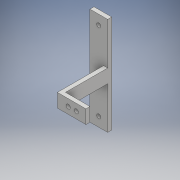
# Autodesk Inventor part: soporteOdroid
Saved by Autodesk Inventor 2017 (Build 210142000, 142)
## iProperties
Part Number: soporteOdroid
Material: Genérico
Document SubType Name: Modeling
Designer: Roberto
Density: 1 g/cm^3
Appearance: Valor por defecto
Author: Roberto
Autodesk Inventor part; units mm, degrees
ref_plane "YZ Plane" through (0, 0, 0) normal (1, 0, 0) x (0, 1, 0)
ref_plane "XZ Plane" through (0, 0, 0) normal (0, 1, 0) x (-1, 0, 0)
ref_plane "XY Plane" through (0, 0, 0) normal (0, 0, 1) x (1, 0, 0)
sketch "Boceto1" plane through (0, 0, 0) normal (0, 1, 0) x (-1, 0, 0)
  circle A0 centre (0.65, -0.45) radius 0.15
  line L0 (0.3, 0) -> (1.3, 0)
  line L1 (1.3, 0) -> (1.3, -1)
  line L2 (1.3, -1) -> (0.3, -1)
  line L3 (0.3, -1) -> (0, -1)
  line L4 (0, -1) -> (0, 0)
  line L5 (0, 0) -> (0.3, 0)
  constraints: 12 end point, 1 centre point
extrude "Extrusión1" add sketch "Boceto1" along normal blind 0.3
sketch "Boceto2" plane through (0, 0, 0) normal (0, -1, 0) x (1, 0, 0)
  line L0 (0, -1) -> (0, 0)
  line L1 (-0.3, -1) -> (0, -1)
  line L2 (0, 0) -> (-0.3, 0)
  line L3 (-0.3, 0) -> (-0.3, -1)
  line L4 (0, 0) -> (0, -1) projected
  line L5 (-0.3, -1) -> (0, -1)
  line L6 (0, -1) -> (0, 0)
  line L7 (0, 0) -> (-0.3, 0)
  line L8 (-0.3, 0) -> (-0.3, -1)
  constraints: 16 end point, 2 parallel, 1 horizontal, 1 perpendicular
extrude "Extrusión2" add sketch "Boceto2" along normal blind 3.4
sketch "Boceto3" plane through (0, 0.3, 0) normal (1, 0, 0) x (0, 0, -1)
  line L0 (1, 0) -> (1, -3.7) projected
  line L1 (0, 0) -> (1, 0) projected
  line L2 (0, 0) -> (0, -3.7) projected
  line L3 (1, -3.7) -> (0, -3.7) projected
  line L4 (0, 0) -> (0, -3.7) projected
  line L5 (0, -3.7) -> (0, -3.4)
  line L6 (0, -3.4) -> (1, -3.4)
  line L7 (1, -3.4) -> (1, -3.7)
  line L8 (1, -3.7) -> (0, -3.7)
  line L9 (0, -3.7) -> (0, -3.4)
  point P0 (0, -0.3)
  dimension "d4" = 0.3
  constraints: 10 end point, 2 parallel, 1 horizontal, 1 perpendicular, 1 point on line
  measures "d4" distance of L2.end L5.end
extrude "Extrusión3" add sketch "Boceto3" along normal blind 1.8 contours L0 L3 L2 L6
sketch "Boceto4" plane through (0, -3.4, 0) normal (0, -1, 0) x (1, 0, 0)
  line L0 (-0.3, 0) -> (1.8, 0) projected
  line L1 (-0.3, 0) -> (-0.3, -1) projected
  line L2 (-0.3, -1) -> (1.8, -1) projected
  line L3 (1.8, 0) -> (1.8, -1) projected
  circle A0 centre (0.5, -0.5) radius 0.15
  circle A1 centre (-6.552, -4.409) radius 0.15
  circle A2 centre (-5.952, -4.409) radius 0.15
  line L4 (0.5, -0.5) -> (1.1, -0.5)
  circle A3 centre (1.1, -0.5) radius 0.15
  point P0 (0, 0)
  dimension "d7" = 0.3
  dimension "d18" = 0.3
  dimension "d19" = 0.3
  dimension "d21" = 0.3
  constraints: 4 centre point, 2 end point, 1 coincident, 1 horizontal
  measures "d7" diameter of A0
  measures "d18" diameter of A1
  measures "d19" diameter of A2
  measures "d21" diameter of A3
extrude "Extrusión4" cut sketch "Boceto4" against normal blind 1 contours A0 | A3
sketch "Boceto6" plane through (0, 0.3, 0) normal (0, 1, 0) x (1, 0, 0)
  line L0 (-1.3, 1) -> (-1.3, 0) projected
  line L1 (-1.3, 0.5) -> (-1.3, 3.4)
  line L2 (0, 3.4) -> (0, -2.4)
  line L3 (-1.3, -2.4) -> (-1.3, 0.5)
  circle A0 centre (-0.65, -2.4) radius 0.15
  circle A1 centre (-0.65, 3.4) radius 0.15
  line L4 (0, 3.4) -> (0, 4.1)
  line L5 (0, 4.1) -> (-1.3, 4.1)
  line L6 (-1.3, 4.1) -> (-1.3, 3.4)
  line L7 (-1.3, -2.4) -> (-1.3, -3.1)
  line L8 (-1.3, -3.1) -> (0, -3.1)
  line L9 (0, -3.1) -> (0, -2.4)
  point P0 (0, 0)
  dimension "d22" = 2.9
  dimension "d23" = 5.8
  dimension "d24" = 1.3
  dimension "d25" = 0.3
  dimension "d26" = 0.3
  dimension "d28" = 0.7
  constraints: 18 end point, 3 perpendicular, 3 point on line, 2 centre point, 2 vertical, 1 collinear, 1 midpoint
  measures "d22" distance of L1.start L1.end
  measures "d23" distance of L2.start L2.end
  measures "d24" distance of L2.end L3.start
  measures "d25" diameter of A0
  measures "d26" diameter of A1
  measures "d28" distance of L3.start L7.end
extrude "Extrusión5" add sketch "Boceto6" against normal blind 0.3
